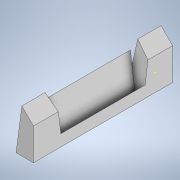
# Autodesk Inventor part: inside-join-half-old
Saved by Autodesk Inventor 2021 (Build 250183000, 183)
## iProperties
Created: 2020-12-10
Part Number: inside-join-half-old
Material: Generic
Document SubType Name: Modeling
Designer: Luke Kamols
Density: 1 g/cm^3
Appearance: Default
Author: Luke Kamols
Autodesk Inventor part; units mm, degrees
ref_plane "YZ Plane" through (0, 0, 0) normal (1, 0, 0) x (0, 1, 0)
ref_plane "XZ Plane" through (0, 0, 0) normal (0, 1, 0) x (-1, 0, 0)
ref_plane "XY Plane" through (0, 0, 0) normal (0, 0, 1) x (1, 0, 0)
sketch "Sketch1" plane through (0, 0, 0) normal (0, 0, 1) x (1, 0, 0)
  line L0 (0, 0) -> (6, 0)
  line L1 (6, 0) -> (6, 11)
  line L2 (6, 11) -> (2, 15)
  line L3 (2, 15) -> (0, 0)
  dimension "d0" = 6
  dimension "d3" = 11
  constraints: 8 end point, 1 horizontal, 1 vertical
  measures "d0" distance of L0.start L0.end
  measures "d3" distance of L0.end L1.end
extrude "Extrusion1" add sketch "Sketch1" along normal blind 10
sketch "Sketch2" plane through (0, 0, 10) normal (0, 0, 1) x (1, 0, 0)
  line L0 (0, 0) -> (6, 0) projected
  line L1 (0, 0) -> (3, 0)
  line L2 (2, 15) -> (0, 0) projected
  line L3 (0, 11) -> (3, 0)
  line L4 (0, 0) -> (-3, 0)
  line L5 (-3, 0) -> (0, 11)
  line L6 (6, 0) -> (6, 4)
  line L7 (6, 0) -> (6, 11) projected
  line L8 (6, 0) -> (5, 0)
  line L9 (5, 0) -> (6, 3.9744)
  dimension "d6" = 3
  dimension "d7" = 11
  dimension "d8" = 3
  dimension "d27" = 4
  dimension "d28" = 1
  constraints: 14 end point, 3 point on line, 1 midpoint
  measures "d6" distance of L0.start L1.end
  measures "d7" distance of L0.start L3.start
  measures "d8" distance of L0.start L4.end
  measures "d27" distance of L0.end L6.end
  measures "d28" distance of L0.end L8.end
extrude "Extrusion2" add sketch "Sketch2" along normal blind 28
sketch "Sketch3" plane through (0, 0, 38) normal (0, 0, 1) x (1, 0, 0)
  line L0 (6, 0) -> (6, 11) projected
  line L1 (0, 0) -> (6, 0) projected
  line L2 (2, 15) -> (0, 0) projected
  line L3 (6, 11) -> (2, 15) projected
extrude "Extrusion3" add sketch "Sketch3" along normal blind 10
sketch "Sketch4" plane through (6, 0, 0) normal (1, 0, 0) x (0, 0, -1)
  line L0 (-10, 0) -> (-38, 0) projected
  line L1 (0, 0) -> (-10, 0) projected
  line L2 (-10, 7.3881) -> (-10, 0) projected
  line L3 (-10, 0) -> (-8, 0)
  line L4 (-8, 0) -> (-8, 15)
  line L5 (0, 15) -> (-10, 15) projected
  line L6 (-10, 0) -> (-8, 15)
  line L7 (-10, 15) -> (-10, 7.3881) projected
  line L8 (-8, 15) -> (-10, 15)
  line L9 (-10, 15) -> (-10, 0)
  dimension "d14" = 2
  constraints: 10 end point, 2 point on line, 1 horizontal, 1 perpendicular, 1 vertical
  measures "d14" distance of L0.start L3.end
extrude "Extrusion4" cut sketch "Sketch4" against normal blind 23.3375 contours L2 L7 L5 L6
sketch "Sketch5" plane through (0, 0, 10) normal (0, 0, -1) x (-1, 0, 0)
  line L0 (3, 0) -> (0, 0) projected
  line L1 (0, 11) -> (3, 0) projected
  line L2 (0, 11) -> (-3, 0) projected
  line L3 (-3, 0) -> (0, 0) projected
  line L4 (-5, 0) -> (-6, 3.9744) projected
  line L5 (-6, 0) -> (-6, 3.9744) projected
  line L6 (-6, 0) -> (-5, 0) projected
extrude "Extrusion5" add sketch "Sketch5" along normal up to surface surface through (6, 15, 8) normal (0, -0.1321637, -0.9912279)
sketch "Sketch6" plane through (6, 0, 38) normal (1, 0, 0) x (0, 0, -1)
  line L0 (0, 3.9744) -> (0, 11) projected
  line L1 (0, 11) -> (-10, 11) projected
  line L2 (-10, 0) -> (-10, 11) projected
  line L3 (0, 11) -> (0, 15) projected
  line L4 (0, 15) -> (-10, 15) projected
  line L5 (-10, 11) -> (-10, 15) projected
  line L6 (0, 11) -> (-10, 11) projected
  line L7 (0, 11) -> (0, 15) projected
  line L8 (0, 0) -> (0, 15)
  line L9 (0, 15) -> (-2, 15)
  line L10 (0, 15) -> (-10, 15) projected
  line L11 (0, 11) -> (0, 0) projected
  line L12 (-2, 15) -> (0, 0)
  line L13 (28.5299, 3.9744) -> (0, 3.9744) projected
  line L14 (38, 0) -> (-10, 0) projected
  line L15 (29.4667, 11) -> (28.5299, 3.9744) projected
  line L16 (38, 0) -> (38, 11) projected
  line L17 (38, 11) -> (29.4667, 11) projected
  point P0 (-2, 15)
  point P1 (-1.4667, 11)
  dimension "d20" = 2
  constraints: 6 end point, 1 point on line, 1 vertical
  measures "d20" distance of L3.end L9.end
extrude "Extrusion6" cut sketch "Sketch6" against normal blind 21.1125 contours L8 L12 L1 L0 | L1 L12 L4 L3
sketch "Sketch7" plane through (0, 0, 38) normal (0, 0, 1) x (1, 0, 0)
  line L0 (3, 0) -> (0, 11) projected
  line L1 (0, 11) -> (-3, 0) projected
  line L2 (-3, 0) -> (0, 0) projected
  line L3 (0, 0) -> (3, 0) projected
  line L4 (6, 3.9744) -> (5, 0) projected
  line L5 (5, 0) -> (6, 0) projected
  line L6 (6, 3.9744) -> (6, 0) projected
extrude "Extrusion7" add sketch "Sketch7" along normal up to surface surface through (6, 0, 38) normal (0, -0.1321637, 0.9912279)
sketch "Sketch9" plane through (0, 0, 0) normal (0, -1, 0) x (1, 0, 0)
  point P0 (0, 0)
body "Solid1"
